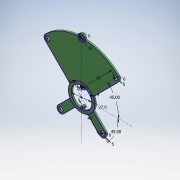
# Autodesk Inventor part: Pok Y-Carriage
Saved by Autodesk Inventor 2018.2 (Build 222227000, 227)
## iProperties
Created: 2018-02-08
Part Number: Pok Y-Carriage
Material: ABS Plastic
Document SubType Name: Modeling
Designer: Moochster
Density: 1.06 g/cm^3
Appearance: Smooth - Dark Forest Green
Author: Moochster
Autodesk Inventor part; units mm, degrees
ref_plane "YZ Plane" through (0, 0, 0) normal (1, 0, 0) x (0, 1, 0)
ref_plane "XZ Plane" through (0, 0, 0) normal (0, 1, 0) x (-1, 0, 0)
ref_plane "XY Plane" through (0, 0, 0) normal (0, 0, 1) x (1, 0, 0)
sketch "Sketch1" plane through (0, 0, 0) normal (0, 1, 0) x (-1, 0, 0)
  circle A0 centre (0, 0) radius 13.95
  line L0 (-1.48, 13.8713) -> (-1.48, 10.9113) construction
  line L1 (-1.48, 10.9113) -> (1.48, 10.9113) construction
  line L2 (1.48, 10.9113) -> (1.48, 13.8713) construction
  line L3 (1.33, 13.8865) -> (1.33, 11.0613)
  line L4 (1.33, 11.0613) -> (-1.33, 11.0613)
  line L5 (-1.33, 11.0613) -> (-1.33, 13.8865)
  line L6 (-1.33, -13.8865) -> (-1.33, -11.0613)
  line L7 (-1.33, -11.0613) -> (1.33, -11.0613)
  line L8 (1.33, -11.0613) -> (1.33, -13.8865)
  arc A1 (15.7257, 8.6547) -> (8.6547, -15.7257) centre (0, 0) ccw
  line L9 (0, 0) -> (0, -53.8283) construction
  line L10 (0, 0) -> (-28.2843, -28.2843) construction
  line L11 (0, 0) -> (-45.9619, 45.9619) construction
  line L12 (0, 0) -> (-69.2668, 0) construction
  circle A2 centre (-28.2843, -28.2843) radius 3
  circle A3 centre (-45.9619, 45.9619) radius 3
  line L13 (-8.6547, -15.7257) -> (-24.7487, -31.8198)
  arc A4 (-31.8198, -24.7487) -> (-24.7487, -31.8198) centre (-28.2843, -28.2843) ccw
  line L14 (-31.8198, -24.7487) -> (-15.7257, -8.6547)
  line L15 (-15.7257, 8.6547) -> (-49.4975, 42.4264)
  arc A5 (-49.4975, 49.4975) -> (-49.4975, 42.4264) centre (-45.9619, 45.9619) ccw
  arc A6 (0, 70) -> (-2.9993, 69.9357) centre (0, 0) ccw
  line L16 (0, 70) -> (0, 0) construction
  circle A7 centre (28.2843, -28.2843) radius 3
  circle A8 centre (45.9619, 45.9619) radius 3
  line L17 (8.6547, -15.7257) -> (24.7487, -31.8198)
  arc A9 (24.7487, -31.8198) -> (31.8198, -24.7487) centre (28.2843, -28.2843) ccw
  line L18 (31.8198, -24.7487) -> (15.7257, -8.6547)
  line L19 (15.7257, 8.6547) -> (49.4975, 42.4264)
  arc A10 (49.4975, 42.4264) -> (49.4975, 49.4975) centre (45.9619, 45.9619) ccw
  arc A11 (49.4975, 49.4975) -> (4.9968, 69.8214) centre (0, 0) ccw
  arc A12 (15.7257, -8.6547) -> (15.7257, 8.6547) centre (0, 0) ccw
  arc A13 (8.6547, -15.7257) -> (15.7257, -8.6547) centre (0, 0) ccw
  circle A14 centre (0, 70) radius 3
  circle A15 centre (0, 70) radius 5
  arc A16 (-2.9993, 69.9357) -> (-4.9968, 69.8214) centre (0, 0) ccw
  arc A17 (2.9993, 69.9357) -> (0, 70) centre (0, 0) ccw
  arc A18 (4.9968, 69.8214) -> (2.9993, 69.9357) centre (0, 0) ccw
  arc A19 (-4.9968, 69.8214) -> (-49.4975, 49.4975) centre (0, 0) ccw
  point P0 (0, 10.9113)
  point P1 (0, 11.0613)
  dimension "d0" = 27.9
  dimension "d1" = 2.96
  dimension "d2" = 2.96
  dimension "d3" = 0.15
  dimension "d4" = 0.15
  dimension "d5" = 0.15
  dimension "d7" = 4
  dimension "d8" = 45
  dimension "d9" = 45
  dimension "d10" = 40
  dimension "d11" = 65
  dimension "d12" = 6
  dimension "d13" = 6
  dimension "d14" = 5
  dimension "d15" = 5
  dimension "d17" = 6
  dimension "d18" = 10
  constraints: 42 point on circle, 40 end point, 20 centre point, 11 symmetric about line, 6 coincident, 6 perpendicular, 4 tangent, 4 vertical, 3 concentric, 3 line through centre, 3 parallel, 3 vertical alignment, 2 midpoint, 1 collinear, 1 horizontal, 5 other
  measures "d0" diameter of A0
  measures "d1" distance of L2.start L2.end
  measures "d2" distance of L0.end L2.start
  measures "d3" distance between parallel lines of L2 L3
  measures "d4" distance between parallel lines of L1 L4
  measures "d5" distance between parallel lines of L0 L5
  measures "d7" radial gap between concentric circles of A1 A0
  measures "d8" angle of L11 L12
  measures "d9" angle of L10 L12
  measures "d10" distance of L9.start L10.end
  measures "d11" distance of L9.start L11.end
  measures "d12" diameter of A2
  measures "d13" diameter of A3
  measures "d14" radius of A4
  measures "d15" radius of A5
  measures "d17" diameter of A14
  measures "d18" diameter of A15
extrude "Extrusion1" add sketch "Sketch1" along normal blind 2.5 contours A12 A13 A1 | A1 L15 A5 A19 A15 A11 A10 L19 | L18 A9 L17 A13 | A1 L13 A4 L14 | A18 A14 A16 A15 | A15 A16 A14 A18
extrude "Extrusion2" add sketch "Sketch1" along normal blind 5 contours L3 L4 L5 A0 | A0 L6 L7 L8
body "Solid1"
